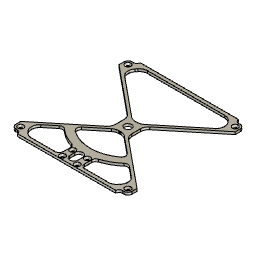
frame-motor (Autodesk Fusion 360 design; units mm, degrees)
Autodesk Fusion 360 part; units mm, degrees
sketch "Sketch1" plane through (0, 0, 0) normal (0, 0, 1) x (1, 0, 0)
  line L0 (0, 0) -> (150, 0)
  line L1 (150, 0) -> (150, 150)
  line L2 (150, 150) -> (0, 150)
  line L3 (0, 150) -> (0, 0)
  dimension "d1" = 150
  dimension "d2" = 150
  constraint horizontal L0
  constraint vertical L1
  constraint horizontal L2
  constraint vertical L3
  constraint coincident L0.start L3.end
  measures "d1" distance of L0.start L0.end
  measures "d2" distance of L0.start L2.end
extrude "Extrude1" add sketch "Sketch1" along normal blind 3
sketch "Sketch2" plane through (0, 0, 3) normal (0, 0, 1) x (-1, 0, 0)
  line L0 (0, -150) -> (0, 0)
  line L1 (0, 0) -> (-150, 0)
  line L2 (-150, 0) -> (-150, -150)
  line L3 (-150, -150) -> (0, -150)
  arc A0 (-4, -9) -> (-9, -4) centre (-9, -9) ccw
  line L4 (0, 0) -> (-15, 0)
  line L5 (-11, -4) -> (-9, -4)
  line L6 (-4, -9) -> (-4, -15)
  line L7 (-4, -15) -> (0, -15)
  line L8 (0, 0) -> (0, -15)
  arc A1 (-15, 0) -> (-11, -4) centre (-11, 0) ccw
  point P0 (-15, 0)
  point P1 (-15, -4)
  point P2 (-9, -4)
  point P3 (-4, -9)
  point P4 (-4, -15)
  point P5 (0, -15)
  dimension "d8" = 15
  dimension "d11" = 5
  dimension "d12" = 4
  dimension "d13" = 4
  dimension "d14" = 15
  dimension "d181" = 4
  constraint coincident L1 P0
  constraint coincident L0 P5
  constraint coincident P2 A0.end
  constraint coincident P3 A0.start
  constraint coincident L0.end L1.start
  constraint coincident P0 L4.end
  constraint tangent A0 L5
  constraint coincident P4 L6.end
  constraint tangent A0 L6
  constraint coincident P5 L7.end
  constraint perpendicular L0 L7
  constraint tangent L5 A1
  measures "d8" distance of L0.end L4.end
  measures "d11" radius of A0
  measures "d12" distance of P0 P1
  measures "d13" distance of P4 P5
  measures "d14" distance of L0.end P5
  measures "d181" radius of A1
sketch "Sketch3" plane through (0, 0, 3) normal (0, 0, 1) x (-1, 0, 0)
  line L0 (-150, -150) -> (0, -150)
  line L1 (0, -150) -> (0, 0)
  line L2 (0, 0) -> (-150, 0)
  line L3 (-150, 0) -> (-150, -150)
  line L4 (0, -75) -> (-65, -75)
  line L5 (-65, -75) -> (-65, -65)
  line L6 (-65, -65) -> (-4, -15)
  line L7 (-4, -15) -> (0, -15)
  line L8 (0, -15) -> (0, -75)
  point P0 (0, -75)
  point P1 (-65, -75)
  point P2 (-65, -65)
  point P3 (0, -15)
  dimension "d25" = 65
  dimension "d27" = 10
  dimension "d50" = 4
  dimension "d51" = 15
  dimension "d52" = 4
  constraint midpoint L1 P0
  constraint coincident P0 L4.start
  constraint coincident P1 L4.end
  constraint perpendicular L1 L4
  constraint coincident P2 L5.end
  constraint perpendicular L4 L5
  constraint coincident L1 P3
  constraint coincident P3 L7.end
  measures "d25" distance of P0 P1
  measures "d27" distance of P1 P2
  measures "d50" horizontal distance of L1.end L6.end
  measures "d51" vertical distance of L1.end L6.end
  measures "d52" distance of L6.end P3
sketch "Sketch4" plane through (0, 0, 3) normal (0, 0, 1) x (-1, 0, 0)
  line L0 (-150, -150) -> (0, -150)
  line L1 (0, 0) -> (-150, 0)
  line L2 (-70, -65) -> (-75, -65)
  line L3 (-75, -65) -> (-75, -4)
  line L4 (-75, -4) -> (-23, -4)
  line L5 (-150, 0) -> (-150, -150)
  line L6 (0, -150) -> (0, 0)
  line L7 (-11.9809, -17.4433) -> (-23, -4)
  line L8 (-11.9809, -17.4433) -> (-70, -65)
  line L9 (-65, -65) -> (-4, -15)
  point P0 (-70, -65)
  point P1 (-75, -65)
  point P2 (-23, -4)
  point P3 (-75, -4)
  point P4 (-11.9809, -17.4433)
  point P5 (-65, -65)
  dimension "d37" = 75
  dimension "d38" = 65
  dimension "d40" = 4
  dimension "d42" = 75
  dimension "d43" = 4
  dimension "d60" = 5
  constraint coincident P0 L2.start
  constraint coincident P1 L2.end
  constraint coincident P3 L3.end
  constraint coincident P2 L4.end
  constraint coincident P4 L7.start
  constraint parallel L8 L9
  constraint perpendicular L7 L8
  measures "d37" horizontal distance of L1.start P1
  measures "d38" vertical distance of L1.start P1
  measures "d40" distance of L1 P2
  measures "d42" horizontal distance of L1.start P3
  measures "d43" distance of L1 P3
  measures "d60" distance of P0 L9.start
ref_plane "WorkPlane2" through (0, 75, 0) normal (0, 1, 0) x (0, 0, 1)
ref_plane "WorkPlane1" through (75, 0, 0) normal (1, 0, 0) x (0, 1, 0)
extrude "Extrude5" cut sketch "Sketch3" sketch "Sketch4" sketch "Sketch2" against normal blind 3 contours L1 L4 L5 L6 L7 L8 of sketch 2 contours L2 L3 L4 L7 L8 of sketch 3 contours L0 L1 A0 L4 L5 L6 L7 L8 A1
fillet "Fillet1" radius 10 4 edges at (23, 4, 1.5) (11.9809, 17.4433, 1.5) (70, 65, 1.5) (65, 65, 1.5)
sketch "Sketch5" plane through (0, 0, 3) normal (0, 0, 1) x (-1, 0, 0)
  line L0 (0, 0) -> (0, -15)
  point P0 (-9.5, -9.5)
  dimension "d67" = 9.5
  dimension "d68" = 9.5
  measures "d67" vertical distance of P0 L0.start
  measures "d68" distance of P0 L0
hole "Hole1" at (9.5, 9.5, 3) direction (0, 0, -1) diameter 3.2 depth 3 tip angle 180 countersink diameter 7 countersink angle 90
mirror "Mirror11" about plane through (75, 0, 0) normal (1, 0, 0) of "Extrude5", "Fillet1", "Hole1"
mirror "Mirror12" about plane through (0, 75, 0) normal (0, 1, 0) of "Extrude5", "Fillet1", "Hole1", "Mirror11"
sketch "Sketch6" plane through (0, 0, 3) normal (0, 0, 1) x (-1, 0, 0)
  line L0 (0, -15) -> (0, -75)
  arc A0 (-41.3577, -43.6281) -> (-75, -29) centre (-75, -75) ccw
  line L1 (-75, -75) -> (-41.3577, -43.6281) construction
  line L2 (-75, -75) -> (-75, -29) construction
  line L3 (-75, -75) -> (-34.7755, -37.4901) construction
  line L4 (-75, -75) -> (-75, -20) construction
  line L5 (-41.3577, -43.6281) -> (-34.7755, -37.4901)
  line L6 (-75, -29) -> (-75, -20)
  line L7 (-62, -21.5584) -> (-62, -4)
  line L8 (-62, -4) -> (-70, -4)
  line L9 (-70, -4) -> (-70, -20.2277)
  arc A1 (-34.7755, -37.4901) -> (-62, -21.5584) centre (-75, -75) ccw
  arc A2 (-70, -20.2277) -> (-75, -20) centre (-75, -75) ccw
  point P0 (-75, -75)
  point P1 (-75, -29)
  point P2 (-75, -20)
  point P3 (-70, -4)
  point P4 (-62, -4)
  dimension "d78" = 75
  dimension "d79" = 75
  dimension "d80" = 46
  dimension "d83" = 55
  dimension "d84" = 75
  dimension "d85" = 75
  dimension "d86" = 47
  dimension "d87" = 47
  dimension "d88" = 5
  dimension "d89" = 8
  dimension "d103" = 4
  constraint coincident P1 A0.end
  constraint coincident P0 A0.centre
  constraint coincident P2 L4.end
  constraint coincident L9.end A1
  constraint coincident L7.start A1.end
  constraint coincident P4 L7.end
  constraint coincident P3 L8.end
  constraint horizontal L8
  constraint coincident L9.end A2.start
  constraint perpendicular L8 L9
  constraint concentric A1 A2
  constraint parallel L7 L9
  measures "d78" vertical distance of P0 origin
  measures "d79" horizontal distance of P0 origin
  measures "d80" distance of P0 A0.end
  measures "d83" distance of P0 P2
  measures "d84" distance of P1 L0
  measures "d85" distance of P2 L0
  measures "d86" angle of L1 L2
  measures "d87" angle of L3 L4
  measures "d88" horizontal distance of P2 P3
  measures "d89" distance of P3 P4
  measures "d103" vertical distance of origin P4
extrude "Extrude6" add sketch "Sketch6" against normal blind 3
sketch "Sketch8" plane through (0, 0, 3) normal (0, 0, 1) x (-1, 0, 0)
  line L0 (0, 0) -> (-150, 0)
  point P0 (-66, -4)
  point P1 (-66, -16.5)
  point P2 (-75, -4)
  dimension "d105" = 9
  dimension "d106" = 9
  dimension "d107" = 4
  dimension "d108" = 12.5
  measures "d105" distance of P0 P2
  measures "d106" horizontal distance of P1 P2
  measures "d107" distance of P0 L0
  measures "d108" distance of P0 P1
hole "Hole2" at (66, 16.5, 3) at (66, 4, 3) direction (0, 0, -1) diameter 3.2 depth 3.3 tip angle 180 countersink diameter 7 countersink angle 90
mirror "Mirror14" about plane through (75, 0, 0) normal (1, 0, 0) of "Extrude6", "Hole2"
sketch "Sketch10" plane through (0, 0, 3) normal (0, 0, 1) x (-1, 0, 0)
  point P0 (-75, -75)
  dimension "d126" = 75
  dimension "d127" = 75
  measures "d126" horizontal distance of P0 origin
  measures "d127" vertical distance of P0 origin
hole "Hole4" at (75, 75, 3) direction (0, 0, -1) diameter 9 depth 3 tip angle 180
fillet "Fillet10" radius 5 12 edges at (35.5036, 36.7242, 1.5) (62, 21.5584, 1.5) (62, 4, 1.5) (42.493, 42.4532, 1.5) (107.507, 42.4532, 1.5) (114.4964, 36.7242, 1.5) (88, 21.5584, 1.5) (70, 20.2277, 1.5) (80, 20.2277, 1.5) (80, 4, 1.5) (70, 4, 1.5) (88, 4, 1.5)
equation "d1 = length_cube"
equation "d2 = length_cube"
equation "length_cube = 150 mm"
equation "thickness = 3 mm"
equation "d5 = thickness"
equation "length_cornerstone = 15 mm"
equation "d8 = length_cornerstone"
equation "distance_corner_cornerstone = 4 mm"
equation "fillet_cornerstone = 5 mm"
equation "d11 = fillet_cornerstone"
equation "d12 = distance_corner_cornerstone"
equation "d13 = distance_corner_cornerstone"
equation "d14 = length_cornerstone"
equation "d17 = length_cube / 2"
equation "d20 = length_cube / 2"
equation "height_centerpiece = 20 mm"
equation "width_centerpiece = 20 mm"
equation "d25 = ( length_cube - width_centerpiece ) / 2"
equation "d27 = height_centerpiece / 2"
equation "d37 = length_cube / 2"
equation "d38 = ( length_cube - height_centerpiece ) / 2"
equation "d40 = distance_corner_cornerstone"
equation "d42 = length_cube / 2"
equation "d43 = distance_corner_cornerstone"
equation "d50 = distance_corner_cornerstone"
equation "d51 = length_cornerstone"
equation "d52 = distance_corner_cornerstone"
equation "d53 = -thickness"
equation "d67 = ( length_cornerstone - distance_corner_cornerstone ) / 2 + distance_corner_cornerstone"
equation "d68 = ( length_cornerstone - distance_corner_cornerstone ) / 2 + distance_corner_cornerstone"
equation "d78 = length_cube / 2"
equation "d79 = length_cube / 2"
equation "d80 = radius_inner_wheel"
equation "radius_inner_wheel = 46 mm"
equation "radius_outer_wheel = 55 mm"
equation "d83 = radius_outer_wheel"
equation "d84 = length_cube / 2"
equation "d85 = length_cube / 2"
equation "d93 = -thickness"
equation "d103 = distance_corner_cornerstone"
equation "d107 = distance_corner_cornerstone"
equation "d126 = length_cube / 2"
equation "d127 = length_cube / 2"
equation "d181 = distance_corner_cornerstone"
